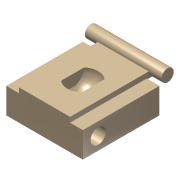
# Autodesk Inventor part: Rocker Box Base
Saved by Autodesk Inventor 2014 (Build 180170000, 170)
## iProperties
Created: 2013-05-18
Part Number: Rocker Box Base
Material: Generic
Document SubType Name: Modeling
Designer: richard
Density: 1 g/cm^3
Appearance: Smooth - Off-White
Author: richard
Autodesk Inventor part; units mm, degrees
ref_plane "YZ Plane" through (0, 0, 0) normal (1, 0, 0) x (0, 1, 0)
ref_plane "XZ Plane" through (0, 0, 0) normal (0, 1, 0) x (-1, 0, 0)
ref_plane "XY Plane" through (0, 0, 0) normal (0, 0, 1) x (1, 0, 0)
sketch "Sketch1" plane through (0, 0, 0) normal (0, 0, 1) x (1, 0, 0)
  line L0 (-37.5, 25) -> (-37.5, 0)
  line L1 (-37.5, 0) -> (37.5, 0)
  line L2 (37.5, 0) -> (37.5, 25)
  line L3 (37.5, 25) -> (25, 25)
  line L4 (25, 25) -> (25, 30)
  line L5 (25, 30) -> (-25, 30)
  line L6 (-25, 30) -> (-25, 25)
  line L7 (-25, 25) -> (-37.5, 25)
  line L8 (0, 0) -> (0, 30) construction
  dimension "d0" = 75
  dimension "d1" = 50
  dimension "d2" = 25
  dimension "d3" = 30
  constraints: 18 end point, 6 parallel, 2 midpoint, 2 perpendicular, 1 coincident, 1 collinear, 1 vertical, 1 other
  measures "d0" distance of L0.end L1.end
  measures "d1" distance of L4.end L5.end
  measures "d2" distance between parallel lines of L7 L1
  measures "d3" distance between parallel lines of L5 L1
extrude "Extrusion1" add sketch "Sketch1" along normal blind 75
sketch "Sketch2" plane through (-25, 30, 0) normal (0, 1, 0) x (1, 0, 0)
  line L0 (0, 0) -> (0, -75) projected
  line L1 (50, 0) -> (50, -75) projected
  line L2 (0, -37.5) -> (50, -37.5)
  line L3 (15, -37.5) -> (15, -26.3197)
  line L4 (35, -26.3197) -> (35, -37.5)
  line L5 (25, -37.5) -> (25, -22.5) construction
  arc A0 (35, -26.3197) -> (15, -26.3197) centre (25, -37.5) ccw
  point P0 (25, 0)
  dimension "d6" = 15
  dimension "d7" = 20
  constraints: 8 end point, 3 midpoint, 3 point on circle, 2 perpendicular, 2 point on line, 1 centre point, 1 coincident, 1 other
  measures "d6" radius of A0
  measures "d7" distance between parallel lines of L4 L3
revolve "Revolution1" cut sketch "Sketch2" angle 360 about axis through (-25, 30, 37.5) along (1, 0, 0)
sketch "Sketch3" plane through (37.5, 0, 0) normal (1, 0, 0) x (0, 0, -1)
  line L0 (0, 25) -> (-75, 25) projected
  line L1 (-75, 0) -> (-75, 25) projected
  line L2 (0, 0) -> (-75, 0) projected
  line L3 (-60, 25) -> (-60, 0) construction
  point P0 (-60, 12.5)
  dimension "d9" = 15
  constraints: 2 end point, 2 point on line, 1 midpoint, 1 perpendicular
  measures "d9" distance between parallel lines of L1 L3
hole "Hole1" at (37.5, 12.5, 60) direction (-1, 0, 0) diameter 15 end through all
sketch "Sketch4" plane through (0, 0, 0) normal (1, 0, 0) x (0, 1, 0)
  circle A0 centre (30, -8) radius 6
  line L0 (30, 0) -> (30, 75) projected
  line L1 (30, 0) -> (30, -2)
  line L2 (24, -8) -> (24, 0)
  line L3 (30, 0) -> (24, 0)
  point P0 (0, 0)
  dimension "d17" = 12
  dimension "d18" = 2
  constraints: 6 end point, 2 point on circle, 1 centre point, 1 collinear, 1 parallel, 1 perpendicular, 1 point on line, 1 tangent
  measures "d17" diameter of A0
  measures "d18" distance of L0.start L1.end
extrude "Extrusion2" add sketch "Sketch4" along normal mid plane 50 contours A0 L2 L3 L1
extrude "Extrusion3" add sketch "Sketch4" along normal mid plane 75 contours A0
fillet "Fillet1" radius 2 1 edges at (0, 24, 0)
body "Solid1"
